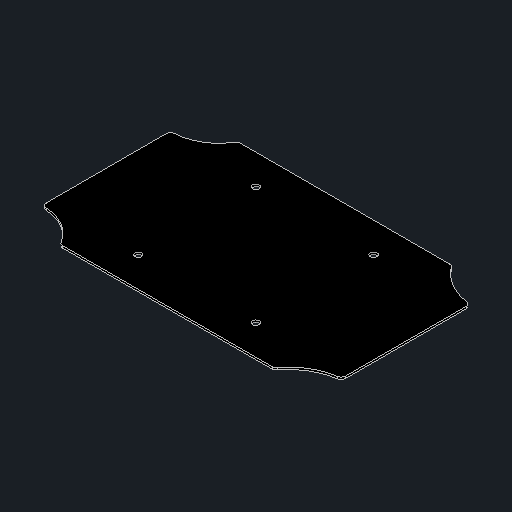
# Autodesk Inventor part: Infrared&ControllerPCB
Saved by Autodesk Inventor 2025.2 (Build 292293000, 293)
## iProperties
Created: 2023-02-24
Part Number: Infrared&ControllerPCB
Material: Aluminum 6061
Document SubType Name: Modeling
Designer: Elias Braun
Density: 2.7 g/cm^3
Appearance: Aluminum - Flat
Author: Elias Braun
Autodesk Inventor part; units mm, degrees
ref_plane "YZ Plane" through (0, 0, 0) normal (1, 0, 0) x (0, 1, 0)
ref_plane "XZ Plane" through (0, 0, 0) normal (0, 1, 0) x (-1, 0, 0)
ref_plane "XY Plane" through (0, 0, 0) normal (0, 0, 1) x (1, 0, 0)
sketch "Sketch3" plane through (0, 0, 0) normal (0, 1, 0) x (-1, 0, 0)
  line L0 (-27.5, -27.5) -> (27.5, -27.5) construction
  line L1 (27.5, -27.5) -> (27.5, 27.5) construction
  line L2 (27.5, 27.5) -> (-27.5, 27.5) construction
  line L3 (-27.5, 27.5) -> (-27.5, -27.5) construction
  line L4 (-27.5, -27.5) -> (27.5, 27.5) construction
  line L5 (27.5, -27.5) -> (-27.5, 27.5) construction
  circle A0 centre (-27.5, 27.5) radius 1.6
  circle A1 centre (27.5, 27.5) radius 1.6
  circle A2 centre (-27.5, -27.5) radius 1.6
  circle A3 centre (27.5, -27.5) radius 1.6
  circle A4 centre (-67.1751, -42.4264) radius 1.6 construction
  line L6 (-27.5, -27.5) -> (-67.1751, -42.4264) construction
  line L7 (-30, -25.7695) -> (-68.0554, -40.0865) construction
  line L8 (-66.2948, -44.7663) -> (-27.0453, -30) construction
  arc A5 (-68.0554, -40.0865) -> (-66.2948, -44.7663) centre (-67.1751, -42.4264) ccw construction
  circle A6 centre (67.1751, -42.4264) radius 1.6 construction
  line L9 (27.5, -27.5) -> (67.1751, -42.4264) construction
  line L10 (27.0453, -30) -> (66.2948, -44.7663) construction
  line L11 (68.0554, -40.0865) -> (30, -25.7695) construction
  arc A7 (66.2948, -44.7663) -> (68.0554, -40.0865) centre (67.1751, -42.4264) ccw construction
  line L12 (27.5, -27.5) -> (-27.5, -27.5) construction
  line L13 (25, -25) -> (-25, -25) construction
  line L14 (-27.0453, -30) -> (27.0453, -30) construction
  line L15 (-27.5, -27.5) -> (-27.5, 27.5) construction
  line L16 (-25, -25) -> (-25, 25) construction
  line L17 (-30, 25.7695) -> (-30, -25.7695) construction
  circle A8 centre (-67.1751, 42.4264) radius 1.6 construction
  line L18 (-27.5, 27.5) -> (-67.1751, 42.4264) construction
  line L19 (-27.0453, 30) -> (-66.2948, 44.7663) construction
  line L20 (-68.0554, 40.0865) -> (-30, 25.7695) construction
  arc A9 (-66.2948, 44.7663) -> (-68.0554, 40.0865) centre (-67.1751, 42.4264) ccw construction
  line L21 (-27.5, 27.5) -> (27.5, 27.5) construction
  line L22 (-25, 25) -> (25, 25) construction
  line L23 (27.0453, 30) -> (-27.0453, 30) construction
  circle A10 centre (67.1751, 42.4264) radius 1.6 construction
  line L24 (27.5, 27.5) -> (67.1751, 42.4264) construction
  line L25 (34.5998, 27.5) -> (68.0554, 40.0865) construction
  line L26 (66.2948, 44.7663) -> (27.0453, 30) construction
  arc A11 (68.0554, 40.0865) -> (66.2948, 44.7663) centre (67.1751, 42.4264) ccw construction
  line L27 (27.5, -27.5) -> (27.5, 27.5) construction
  line L28 (30, -25.7695) -> (30, 25.7695) construction
  line L29 (25, 25) -> (25, -25) construction
  line L30 (34.5998, 27.5) -> (30, 25.7695) construction
  line L31 (55, 55) -> (-55, -55) construction
  line L32 (-55, 55) -> (55, -55) construction
  circle A12 centre (0, 0) radius 110 construction
  arc A13 (43.0581, -98.5) -> (-43.0581, -98.5) centre (0, 0) ccw construction
  line L33 (0, -107.5) -> (0, -98.5) construction
  line L34 (0, -98.5) -> (0, -73.5) construction
  line L35 (0, -98.5) -> (-43.0581, -98.5) construction
  line L36 (0, -98.5) -> (43.0581, -98.5) construction
  line L37 (43.0581, -98.5) -> (-43.0581, -98.5) construction
  line L38 (-18.0581, -73.5) -> (18.0581, -73.5) construction
  arc A14 (43.0581, -98.5) -> (18.0581, -73.5) centre (18.0581, -98.5) ccw construction
  arc A15 (-18.0581, -73.5) -> (-43.0581, -98.5) centre (-18.0581, -98.5) ccw construction
  line L39 (0, 107.5) -> (0, 97.5) construction
  line L40 (0, 97.5) -> (-22.5, 97.5) construction
  line L41 (-22.5, 97.5) -> (-22.5, 82.5) construction
  line L42 (22.5, 82.5) -> (22.5, 97.5) construction
  line L43 (22.5, 90) -> (-22.5, 90) construction
  line L44 (15, 97.5) -> (-15, 97.5)
  line L45 (-15, 82.5) -> (15, 82.5)
  arc A16 (15, 82.5) -> (15, 97.5) centre (15, 90) ccw
  arc A17 (-15, 97.5) -> (-15, 82.5) centre (-15, 90) ccw
  line L46 (22.5, 82.5) -> (17.5, 82.5) construction
  line L47 (17.5, 82.5) -> (17.5, 77.5) construction
  circle A18 centre (17.5, 77.5) radius 1.6
  circle A19 centre (-17.5, 77.5) radius 1.6
  line L48 (-58.3363, 79.5495) -> (-79.5495, 58.3363) construction
  arc A20 (-47.7297, 68.9429) -> (-58.3363, 79.5495) centre (-53.033, 74.2462) ccw construction
  arc A21 (-79.5495, 58.3363) -> (-68.9429, 47.7297) centre (-74.2462, 53.033) ccw construction
  line L49 (-68.9429, 47.7297) -> (-47.7297, 68.9429) construction
  circle A22 centre (-67.1751, 42.4264) radius 1.6 construction
  circle A23 centre (-42.4264, 67.1751) radius 1.6 construction
  line L50 (-97.5, 15) -> (-97.5, -15)
  arc A24 (-82.5, 15) -> (-97.5, 15) centre (-90, 15) ccw
  arc A25 (-97.5, -15) -> (-82.5, -15) centre (-90, -15) ccw
  line L51 (-82.5, -15) -> (-82.5, 15)
  circle A26 centre (-77.5, -17.5) radius 1.6
  circle A27 centre (-77.5, 17.5) radius 1.6
  line L52 (-79.5495, -58.3363) -> (-58.3363, -79.5495) construction
  arc A28 (-68.9429, -47.7297) -> (-79.5495, -58.3363) centre (-74.2462, -53.033) ccw construction
  arc A29 (-58.3363, -79.5495) -> (-47.7297, -68.9429) centre (-53.033, -74.2462) ccw construction
  line L53 (-47.7297, -68.9429) -> (-68.9429, -47.7297) construction
  circle A30 centre (-42.4264, -67.1751) radius 1.6 construction
  circle A31 centre (-67.1751, -42.4264) radius 1.6 construction
  line L54 (-15, -97.5) -> (15, -97.5)
  arc A32 (-15, -82.5) -> (-15, -97.5) centre (-15, -90) ccw
  arc A33 (15, -97.5) -> (15, -82.5) centre (15, -90) ccw
  line L55 (15, -82.5) -> (-15, -82.5)
  circle A34 centre (17.5, -77.5) radius 1.6
  circle A35 centre (-17.5, -77.5) radius 1.6
  line L56 (58.3363, -79.5495) -> (79.5495, -58.3363) construction
  arc A36 (47.7297, -68.9429) -> (58.3363, -79.5495) centre (53.033, -74.2462) ccw construction
  arc A37 (79.5495, -58.3363) -> (68.9429, -47.7297) centre (74.2462, -53.033) ccw construction
  line L57 (68.9429, -47.7297) -> (47.7297, -68.9429) construction
  circle A38 centre (67.1751, -42.4264) radius 1.6 construction
  circle A39 centre (42.4264, -67.1751) radius 1.6 construction
  line L58 (97.5, -15) -> (97.5, 15)
  arc A40 (82.5, -15) -> (97.5, -15) centre (90, -15) ccw
  arc A41 (97.5, 15) -> (82.5, 15) centre (90, 15) ccw
  line L59 (82.5, 15) -> (82.5, -15)
  circle A42 centre (77.5, 17.5) radius 1.6
  circle A43 centre (77.5, -17.5) radius 1.6
  line L60 (79.5495, 58.3363) -> (58.3363, 79.5495) construction
  arc A44 (68.9429, 47.7297) -> (79.5495, 58.3363) centre (74.2462, 53.033) ccw construction
  arc A45 (58.3363, 79.5495) -> (47.7297, 68.9429) centre (53.033, 74.2462) ccw construction
  line L61 (47.7297, 68.9429) -> (68.9429, 47.7297) construction
  circle A46 centre (42.4264, 67.1751) radius 1.6 construction
  circle A47 centre (67.1751, 42.4264) radius 1.6 construction
  line L62 (58.3363, -58.3363) -> (51.2652, -51.2652) construction
  line L63 (40.6586, -61.8718) -> (61.8718, -40.6586) construction
  arc A48 (40.6586, -61.8718) -> (44.5267, -89.5398) centre (53.033, -74.2462) ccw construction
  arc A49 (89.5398, -44.5267) -> (61.8718, -40.6586) centre (74.2462, -53.033) ccw construction
  line L64 (0, -73.5) -> (0, -66.5) construction
  arc A50 (44.5267, 89.5398) -> (40.6586, 61.8718) centre (53.033, 74.2462) ccw construction
  line L65 (61.8718, 40.6586) -> (40.6586, 61.8718) construction
  arc A51 (61.8718, 40.6586) -> (89.5398, 44.5267) centre (74.2462, 53.033) ccw construction
  arc A52 (-89.5398, 44.5267) -> (-61.8718, 40.6586) centre (-74.2462, 53.033) ccw construction
  line L66 (-40.6586, 61.8718) -> (-61.8718, 40.6586) construction
  arc A53 (-40.6586, 61.8718) -> (-44.5267, 89.5398) centre (-53.033, 74.2462) ccw construction
  arc A54 (-44.5267, -89.5398) -> (-40.6586, -61.8718) centre (-53.033, -74.2462) ccw construction
  line L67 (-61.8718, -40.6586) -> (-40.6586, -61.8718) construction
  arc A55 (-61.8718, -40.6586) -> (-89.5398, -44.5267) centre (-74.2462, -53.033) ccw construction
  arc A56 (89.5398, -44.5267) -> (89.5398, 44.5267) centre (0, 0) ccw construction
  arc A57 (44.5267, 89.5398) -> (-44.5267, 89.5398) centre (0, 0) ccw construction
  arc A58 (-89.5398, 44.5267) -> (-89.5398, -44.5267) centre (0, 0) ccw construction
  line L68 (43.0581, -98.5) -> (48.0581, -98.5) construction
  line L69 (48.0581, -98.5) -> (48.0581, -88.5) construction
  circle A59 centre (48.0581, -88.5) radius 1.6 construction
  circle A60 centre (-48.0581, -88.5) radius 1.6 construction
  line L70 (18.0581, -66.5) -> (-18.0581, -66.5) construction
  arc A61 (17.5, -66.5) -> (43.0581, -59.4724) centre (19.5145, -23.8377) ccw construction
  arc A62 (-44.5267, -58.0038) -> (-18.0581, -66.5) centre (-19.5089, -25.5422) ccw construction
  line L71 (0, -66.5) -> (0, -41.5) construction
  line L72 (0, -41.5) -> (50, -41.5)
  line L73 (0, -41.5) -> (-50, -41.5)
  line L74 (107.5, 0) -> (70, 0) construction
  line L75 (70, 0) -> (70, -30)
  line L76 (70, 0) -> (70, 30)
  line L77 (-70, 0) -> (-70, -30)
  line L78 (-70, 0) -> (-70, 30)
  arc A63 (70, -30) -> (50, -41.5) centre (69.3076, -51.9372) ccw
  arc A64 (-50, -41.5) -> (-70, -30) centre (-72.2179, -56.9986) ccw
  line L79 (0, 0) -> (15.9, 0) construction
  line L80 (0, 41.5) -> (50, 41.5)
  line L81 (0, 41.5) -> (-50, 41.5)
  arc A65 (50, 41.5) -> (70, 30) centre (69.3076, 51.9372) ccw
  arc A66 (-70, 30) -> (-50, 41.5) centre (-72.2179, 56.9986) ccw
  point P0 (-47.3376, -34.9632)
  point P1 (47.3376, -34.9632)
  point P2 (0, -27.5)
  point P3 (-27.5, 0)
  point P4 (-47.3376, 34.9632)
  point P5 (0, 27.5)
  point P6 (47.3376, 34.9632)
  point P7 (27.5, 0)
  point P8 (0, 90)
  point P9 (-45.9619, 70.7107)
  point P10 (-82.5, 17.5)
  point P11 (-70.7107, -45.9619)
  point P12 (-17.5, -82.5)
  point P13 (45.9619, -70.7107)
  point P14 (82.5, -17.5)
  point P15 (70.7107, 45.9619)
  point P16 (35.7159, -76.7698)
  dimension "d50" = 55
  dimension "d51" = 55
  dimension "d52" = 3.2
  dimension "d53" = 3.2
  dimension "d54" = 3.2
  dimension "d55" = 3.2
  dimension "d56" = 5
  dimension "d57" = 5
  dimension "d58" = 5
  dimension "d59" = 5
  dimension "d60" = 110
  dimension "d67" = 220
  dimension "d68" = 215
  dimension "d69" = 9
  dimension "d70" = 25
  dimension "d71" = 10
  dimension "d72" = 22.5
  dimension "d73" = 15
  dimension "d74" = 45
  dimension "d75" = 5
  dimension "d76" = 5
  dimension "d77" = 3.2
  dimension "d78" = 86.1162
  dimension "d79" = 45
  dimension "d80" = 360
  dimension "d81" = 10
  dimension "d82" = 7
  dimension "d83" = 360
  dimension "d84" = 5
  dimension "d85" = 10
  dimension "d86" = 3.2
  dimension "d87" = 25
  dimension "d88" = 50
  dimension "d89" = 50
  dimension "d90" = 37.5
  dimension "d91" = 30
  dimension "d92" = 30
  constraints: 184 end point, 87 point on circle, 67 centre point, 21 point on line, 17 midpoint, 14 tangent, 11 parallel, 10 symmetric about line, 9 coincident, 8 vertical, 7 horizontal, 3 collinear, 3 perpendicular, 162 other
  measures "d50" distance of L0.start L0.end
  measures "d51" distance of L1.end L0.end
  measures "d52" diameter of A0
  measures "d53" diameter of A1
  measures "d54" diameter of A2
  measures "d55" diameter of A3
  measures "d56" diameter of A5
  measures "d57" diameter of A7
  measures "d58" diameter of A9
  measures "d59" diameter of A11
  measures "d60" distance of L31.end L32.start
  measures "d67" diameter of A12
  measures "d68" diameter of A13
  measures "d69" distance of L33.start L33.end
  measures "d70" distance of L33.end L34.end
  measures "d71" distance of L39.start L39.end
  measures "d72" distance of L39.end L40.end
  measures "d73" distance of L40.end L41.end
  measures "d74" distance of L41.end L42.start
  measures "d75" distance of L42.start L46.end
  measures "d76" distance of L46.end L47.end
  measures "d77" diameter of A18
  measures "d78" distance of L36.end L35.end
  measures "d79" distance of L43.start L43.end
  measures "d81" distance of L62.start L62.end
  measures "d82" distance of L34.end L64.end
  measures "d84" distance of L36.end L68.end
  measures "d85" distance of L68.end L69.end
  measures "d86" diameter of A59
  measures "d87" distance of L64.end L71.end
  measures "d88" distance of L71.end L72.end
  measures "d89" distance of L71.end L73.end
  measures "d90" distance of L74.start L74.end
  measures "d91" distance of L74.end L75.end
  measures "d92" distance of L74.end L76.end
extrude "Extrusion3" add sketch "Sketch3" along normal blind 1 contours L73 A64 L77 L78 A66 L81 L80 A65 L76 L75 A63 L72
fillet "Fillet1" radius 2 8 edges at (50, 0.5, 41.5) (70, 0.5, 30) (70, 0.5, -30) (50, 0.5, -41.5) (-50, 0.5, 41.5) (-70, 0.5, 30) (-70, 0.5, -30) (-50, 0.5, -41.5)
body "Solid3"
